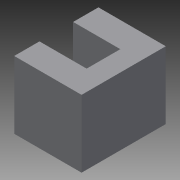
# Autodesk Inventor part: EE-SX1131
Saved by Autodesk Inventor 2014 (Build 180170000, 170)
## iProperties
Created: 2013-05-31
Part Number: EE-SX1131
Material: Generisch
Document SubType Name: Modeling
Designer: hanse
Density: 1 g/cm^3
Appearance: Vorgabe
Author: hanse
Autodesk Inventor part; units mm, degrees
ref_plane "YZ Plane" through (0, 0, 0) normal (1, 0, 0) x (0, 1, 0)
ref_plane "XZ Plane" through (0, 0, 0) normal (0, 1, 0) x (-1, 0, 0)
ref_plane "XY Plane" through (0, 0, 0) normal (0, 0, 1) x (1, 0, 0)
sketch "Skizze1" plane through (0, 0, 0) normal (1, 0, 0) x (0, 1, 0)
  line L0 (0, 0) -> (5, 0)
  line L1 (5, 0) -> (5, 4)
  line L2 (5, 4) -> (0, 4)
  line L3 (0, 4) -> (0, 0)
  dimension "d0" = 5
  dimension "d1" = 4
  constraints: 8 end point, 2 parallel, 1 horizontal, 1 perpendicular
  measures "d0" distance of L1.end L2.end
  measures "d1" distance of L0.end L1.end
extrude "Extrusion1" add sketch "Skizze1" along normal blind 1.2
sketch "Skizze2" plane through (0, 0, 0) normal (-1, 0, 0) x (0, 0, 1)
  line L0 (0, 0) -> (0, 5) projected
  line L1 (4, 0) -> (0, 0) projected
  line L2 (4, 5) -> (4, 0) projected
  line L3 (0, 5) -> (4, 5) projected
  line L4 (4, 3.5) -> (0, 3.5)
  line L5 (4, 1.5) -> (0, 1.5)
  dimension "d4" = 1.5
  dimension "d5" = 1.5
  constraints: 4 end point, 4 point on line, 2 perpendicular
  measures "d4" distance between parallel lines of L5 L1
  measures "d5" distance between parallel lines of L3 L4
extrude "Extrusion2" add sketch "Skizze2" along normal blind 2.8 contours L0 L5 L2 L1 | L0 L3 L2 L4
